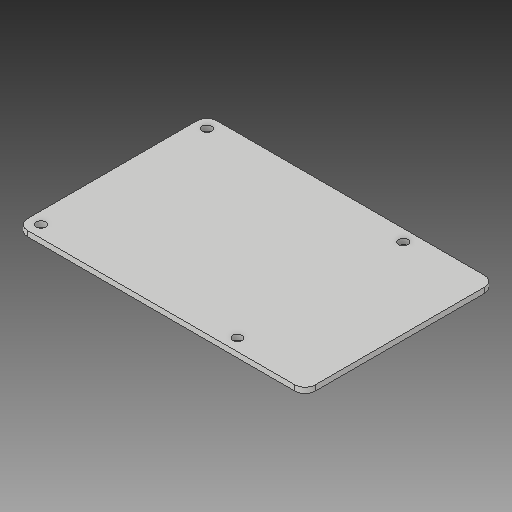
# Autodesk Inventor part: Raspberry-Pi-3B[with_Screen]
Saved by Autodesk Inventor 2017 (Build 210142000, 142)
## iProperties
Created: 2018-04-18
Part Number: Raspberry-Pi-3B[with_Screen]
Material: Generic
Document SubType Name: Modeling
Designer: MtgSaber
Density: 1 g/cm^3
Appearance: Default
Author: MtgSaber
Autodesk Inventor part; units mm, degrees
ref_plane "YZ Plane" through (0, 0, 0) normal (1, 0, 0) x (0, 1, 0)
ref_plane "XZ Plane" through (0, 0, 0) normal (0, 1, 0) x (-1, 0, 0)
ref_plane "XY Plane" through (0, 0, 0) normal (0, 0, 1) x (1, 0, 0)
sketch "Sketch1" plane through (0, 0, 0) normal (0, 1, 0) x (-1, 0, 0)
  line L0 (42.4942, 28.0035) -> (-42.4942, 28.0035) construction
  line L1 (-42.4942, 28.0035) -> (-42.4942, -28.0035) construction
  line L2 (-42.4942, -28.0035) -> (42.4942, -28.0035) construction
  line L3 (42.4942, -28.0035) -> (42.4942, 28.0035) construction
  line L4 (0, -40.0739) -> (0, 40.0739) construction
  line L5 (60.3609, 0) -> (-60.3609, 0) construction
  circle A0 centre (38.989, -24.4983) radius 1.3716
  circle A1 centre (-18.9992, -24.4983) radius 1.3716
  circle A2 centre (-18.9992, 24.4983) radius 1.3716
  circle A3 centre (38.989, 24.4983) radius 1.3716
  line L6 (42.4942, 25.0063) -> (42.4942, -25.0063)
  line L7 (39.497, 28.0035) -> (-39.497, 28.0035)
  line L8 (-42.4942, 25.0063) -> (-42.4942, -25.0063)
  line L9 (-39.497, -28.0035) -> (39.497, -28.0035)
  arc A4 (42.4942, 25.0063) -> (39.497, 28.0035) centre (39.497, 25.0063) ccw
  arc A5 (39.497, -28.0035) -> (42.4942, -25.0063) centre (39.497, -25.0063) ccw
  arc A6 (-42.4942, -25.0063) -> (-39.497, -28.0035) centre (-39.497, -25.0063) ccw
  arc A7 (-39.497, 28.0035) -> (-42.4942, 25.0063) centre (-39.497, 25.0063) ccw
  point P0 (0, 0)
  dimension "d0" = 84.9884
  dimension "d1" = 56.007
  dimension "d2" = 0
  dimension "d3" = 0
  dimension "d4" = 0
  dimension "d5" = 0
  dimension "d6" = 2.7432
  dimension "d7" = 3.5052
  dimension "d8" = 3.5052
  dimension "d9" = 3.5052
  dimension "d10" = 57.9882
  dimension "d11" = 2.9972
  dimension "d12" = 2.9972
  dimension "d13" = 2.9972
  dimension "d14" = 2.9972
  dimension "d15" = 2.9972
  dimension "d16" = 2.9972
  dimension "d17" = 2.9972
  dimension "d18" = 2.9972
  constraints: 16 end point, 9 point on circle, 8 centre point, 4 coincident, 4 tangent, 3 equal radius, 3 perpendicular, 3 point on line, 2 collinear, 2 parallel, 1 horizontal
  measures "d0" distance of L1.end L2.end
  measures "d1" distance of L0.end L1.end
  measures "d2" horizontal distance of A0.centre A3.centre
  measures "d3" horizontal distance of A2.centre A1.centre
  measures "d4" vertical distance of A3.centre A2.centre
  measures "d5" vertical distance of A0.centre A1.centre
  measures "d6" diameter of A0
  measures "d7" distance from line of L0 A3.centre
  measures "d8" distance from line of L3 A3.centre
  measures "d9" distance from line of L2 A0.centre
  measures "d10" distance of A0.centre A1.centre
  measures "d11" distance from line of L8 point (-39.497, 25.006)
  measures "d12" distance from line of L0 point (-39.497, 25.006)
  measures "d13" distance from line of L2 point (-39.497, -25.006)
  measures "d14" distance from line of L1 point (-39.497, -25.006)
  measures "d15" distance from line of L2 point (39.497, -25.006)
  measures "d16" distance from line of L3 point (39.497, -25.006)
  measures "d17" distance from line of L0 point (39.497, 25.006)
  measures "d18" distance from line of L3 point (39.497, 25.006)
extrude "Extrusion1" add sketch "Sketch1" along normal blind 1.6002
body "Solid1"
